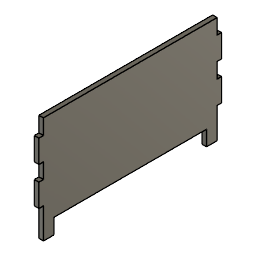
Muur Lang (Autodesk Fusion 360 design; units mm, degrees)
part number: 2026-03-12-08-56-11-008
Autodesk Fusion 360 part; units mm, degrees
sketch "Sketch1" plane through (0, 0, 0) normal (0, 0, 1) x (1, 0, 0)
  line L0 (36.0863, 68.8405) -> (39.0863, 68.8405)
  line L1 (39.0863, 68.8405) -> (39.0863, -51.1595)
  line L2 (39.0863, -51.1595) -> (36.0863, -51.1595)
  line L3 (36.0863, -51.1595) -> (36.0863, 68.8405)
  dimension "d1" = 3
  dimension "d2" = 120
  constraint horizontal L0
  constraint vertical L1
  constraint horizontal L2
  constraint vertical L3
  measures "d1" distance of L1.end L2.end
  measures "d2" distance of L0.end L1.end
extrude "Extrude1" add sketch "Sketch1" along normal blind 70
sketch "Sketch2" plane through (36.0863, 0, 0) normal (-1, 0, 0) x (0, -1, 0)
  line L0 (-68.8405, 0) -> (51.1595, 0)
  line L1 (51.1595, 0) -> (51.1595, 70)
  line L2 (51.1595, 70) -> (-68.8405, 70)
  line L3 (-68.8405, 70) -> (-68.8405, 0)
  line L4 (-58.8405, 0) -> (41.1595, 0)
  line L5 (41.1595, 0) -> (41.1595, 10)
  line L6 (41.1595, 10) -> (-58.8405, 10)
  line L7 (-58.8405, 10) -> (-58.8405, 0)
  dimension "d5" = 10
  dimension "d6" = 100
  dimension "d7" = 10
  constraint horizontal L4
  constraint vertical L5
  constraint horizontal L6
  constraint vertical L7
  constraint coincident L0 L4.start
  measures "d5" distance of L0.start L4.start
  measures "d6" distance of L4.start L4.end
  measures "d7" distance of L4.start L6.end
extrude "Extrude2" cut sketch "Sketch2" against normal blind 15 contours L0 L4 L5 L6 L7
sketch "Sketch3" plane through (36.0863, 0, 0) normal (-1, 0, 0) x (0, -1, 0)
  line L0 (41.1595, 10) -> (41.1595, 0)
  line L1 (41.1595, 0) -> (51.1595, 0)
  line L2 (51.1595, 0) -> (51.1595, 70)
  line L3 (51.1595, 70) -> (-68.8405, 70)
  line L4 (-68.8405, 70) -> (-68.8405, 0)
  line L5 (-68.8405, 0) -> (-58.8405, 0)
  line L6 (-58.8405, 0) -> (-58.8405, 10)
  line L7 (-58.8405, 10) -> (41.1595, 10)
  line L8 (-81.9379, 60) -> (81.0278, 60) construction
  line L9 (-84.1729, 45) -> (76.1854, 45) construction
  line L10 (-82.6829, 35) -> (77.4892, 35) construction
  line L11 (-85.6629, 20) -> (78.0479, 20) construction
  line L12 (-65.8405, 82.86) -> (-65.8405, -11.3972) construction
  line L13 (48.1595, 79.5603) -> (48.1595, -14.1231) construction
  line L14 (-65.8405, 60) -> (-65.8405, 45) construction
  line L15 (-65.8405, 45) -> (-68.8405, 45) construction
  line L16 (-68.8405, 35) -> (-65.8405, 35) construction
  line L17 (-65.8405, 35) -> (-65.8405, 20) construction
  line L18 (-65.8405, 20) -> (-68.8405, 20) construction
  line L19 (51.1595, 20) -> (48.1595, 20) construction
  line L20 (48.1595, 20) -> (48.1595, 35) construction
  line L21 (48.1595, 35) -> (51.1595, 35) construction
  line L22 (51.1595, 35) -> (51.1595, 20) construction
  line L23 (51.1595, 45) -> (48.1595, 45) construction
  line L24 (48.1595, 60) -> (51.1595, 60) construction
  line L25 (51.1595, 60) -> (51.1595, 45) construction
  line L26 (-65.8405, 45) -> (-68.8405, 45)
  line L27 (-65.8405, 60) -> (-68.8405, 60)
  line L28 (-68.8405, 60) -> (-68.8405, 70)
  line L29 (-68.8405, 70) -> (-65.8405, 70)
  line L30 (-65.8405, 70) -> (-65.8405, 60)
  line L31 (-65.8405, 35) -> (-68.8405, 35)
  line L32 (-68.8405, 35) -> (-68.8405, 45)
  line L33 (-68.8405, 45) -> (-65.8405, 45)
  line L34 (-65.8405, 45) -> (-65.8405, 35)
  line L35 (-65.8405, 0) -> (-68.8405, 0)
  line L36 (-68.8405, 0) -> (-68.8405, 20)
  line L37 (-68.8405, 20) -> (-65.8405, 20)
  line L38 (-65.8405, 20) -> (-65.8405, 0)
  line L39 (51.1595, 0) -> (48.1595, 0)
  line L40 (48.1595, 0) -> (48.1595, 20)
  line L41 (48.1595, 20) -> (51.1595, 20)
  line L42 (51.1595, 20) -> (51.1595, 0)
  line L43 (51.1595, 35) -> (48.1595, 35)
  line L44 (48.1595, 35) -> (48.1595, 45)
  line L45 (48.1595, 45) -> (51.1595, 45)
  line L46 (51.1595, 45) -> (51.1595, 35)
  line L47 (51.1595, 60) -> (48.1595, 60)
  line L48 (48.1595, 60) -> (48.1595, 70)
  line L49 (48.1595, 70) -> (51.1595, 70)
  line L50 (51.1595, 70) -> (51.1595, 60)
  dimension "d10" = 10
  dimension "d11" = 15
  dimension "d12" = 10
  dimension "d13" = 15
  dimension "d14" = 3
  dimension "d15" = 3
  constraint perpendicular L2 L8
  constraint perpendicular L4 L9
  constraint horizontal L10
  constraint perpendicular L6 L11
  constraint perpendicular L5 L12
  constraint vertical L13
  constraint vertical L14
  constraint horizontal L15
  constraint coincident L12 L14.end
  constraint coincident L9 L14.end
  constraint horizontal L16
  constraint vertical L17
  constraint horizontal L18
  constraint coincident L11 L17.end
  constraint coincident L12 L17.end
  constraint coincident L10 L16.start
  constraint coincident L4 L16.start
  constraint horizontal L19
  constraint vertical L20
  constraint horizontal L21
  constraint vertical L22
  constraint coincident L13 L20.end
  constraint coincident L10 L20.end
  constraint coincident L11 L19.start
  constraint coincident L2 L19.start
  constraint horizontal L23
  constraint horizontal L24
  constraint vertical L25
  constraint coincident L13 L24.start
  constraint coincident L8 L24.start
  constraint coincident L9 L23.start
  constraint coincident L2 L23.start
  constraint horizontal L26
  constraint horizontal L27
  constraint vertical L28
  constraint horizontal L29
  constraint vertical L30
  constraint coincident L3.end L4.start
  constraint horizontal L31
  constraint vertical L32
  constraint horizontal L33
  constraint vertical L34
  constraint horizontal L35
  constraint vertical L36
  constraint horizontal L37
  constraint vertical L38
  constraint coincident L12 L35.start
  constraint coincident L5 L35.start
  constraint horizontal L39
  constraint vertical L40
  constraint horizontal L41
  constraint vertical L42
  constraint coincident L1.end L2.start
  constraint horizontal L43
  constraint vertical L44
  constraint horizontal L45
  constraint vertical L46
  constraint horizontal L47
  constraint vertical L48
  constraint horizontal L49
  constraint vertical L50
  constraint coincident L3 L48.end
  constraint coincident L13 L48.end
  measures "d10" distance of L3 L8
  measures "d11" distance of L8 L9
  measures "d12" distance of L9 L10
  measures "d13" distance of L10 L11
  measures "d14" distance of L4 L12
  measures "d15" distance of L2 L13
extrude "Extrude3" cut sketch "Sketch3" against normal blind 30 contours L1 L2 L39 L40 L41 L42 | L4 L5 L35 L36 L37 L38 | L2 L43 L44 L45 L46 | L4 L26 L31 L32 L33 L34 | L2 L3 L47 L48 L49 L50 | L3 L4 L27 L28 L29 L30
